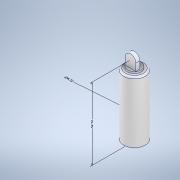
# Autodesk Inventor part: Arm1
Saved by Autodesk Inventor 2022 (Build 260153000, 153)
## iProperties
Created: 2021-10-29
Part Number: Arm1
Material: Aluminum 6061
Document SubType Name: Modeling
Designer: Mark Maara
Density: 2.7 g/cm^3
Appearance: Aluminum - Flat
Mass: 8319.53 g
Surface Area: 2297.12 cm^2
Volume: 3081.31 cm^3
Author: Mark Maara
Autodesk Inventor part; units mm, degrees
ref_plane "YZ Plane" through (0, 0, 0) normal (1, 0, 0) x (0, 1, 0)
ref_plane "XZ Plane" through (0, 0, 0) normal (0, 1, 0) x (-1, 0, 0)
ref_plane "XY Plane" through (0, 0, 0) normal (0, 0, 1) x (1, 0, 0)
sketch "Sketch1" plane through (0, 0, 0) normal (0, 1, 0) x (-1, 0, 0)
  circle A0 centre (0, 0) radius 60
  circle A1 centre (0, 0) radius 30
  dimension "d0" = 120
  dimension "d3" = 60
  constraints: 2 centre point, 2 coincident
  measures "d0" diameter of A0
  measures "d3" diameter of A1
extrude "Extrusion1" add sketch "Sketch1" along normal blind 350
sketch "Sketch2" plane through (0, 350, 0) normal (0, 1, 0) x (1, 0, 0)
  circle A0 centre (0, 0) radius 37.5
  dimension "d7" = 75
  constraints: 1 centre point, 1 coincident
  measures "d7" diameter of A0
extrude "Extrusion2" add sketch "Sketch2" along normal blind 10
sketch "Sketch4" plane through (0, 360, 0) normal (0, 1, 0) x (1, 0, 0)
  point P0 (0, 0)
sketch "Sketch5" plane through (0, 0, 0) normal (0, 0, 1) x (1, 0, 0)
  line L0 (37.5, 360) -> (-37.5, 360) projected
  line L1 (0, 360) -> (0, 400)
  circle A0 centre (0, 400) radius 30
  line L2 (30, 400) -> (30, 360)
  line L3 (-30, 400) -> (-30, 360)
  line L4 (-30, 360) -> (30, 360)
  point P0 (0, 0)
  dimension "d13" = 40
  dimension "d14" = 60
  constraints: 8 end point, 3 perpendicular, 2 point on circle, 2 point on line, 2 tangent, 1 centre point, 1 coincident, 1 midpoint, 1 vertical
  measures "d13" distance of L1.start L1.end
  measures "d14" diameter of A0
extrude "Extrusion4" add sketch "Sketch5" along normal blind 22
fillet "Fillet1" radius 10 2 edges at (60, 350, 0) (60, 0, 0)
ref_plane "Work Plane1" through (0, 175, 0) normal (0, -1, 0) x (1, 0, 0)
sketch "Sketch6" plane through (0, 175, 0) normal (0, -1, 0) x (1, 0, 0)
  circle A0 centre (0, 0) radius 57.5
  dimension "d23" = 115
  constraints: 1 centre point, 1 coincident
  measures "d23" diameter of A0
extrude "Extrusion5" cut sketch "Sketch6" along normal mid plane 300
shell "Shell1" thickness 6.5 removed faces 0
body "Solid1"
